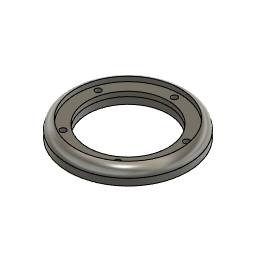
rear_speaker_adapter v3 (Autodesk Fusion 360 design; units mm, degrees)
Autodesk Fusion 360 part; units mm, degrees
note: some values were not read from the file. Chosen so that the rebuilt part matches the saved one: which face or edge a step refers to.
sketch "Sketch1" plane through (0, 0, 0) normal (0, 1, 0) x (1, 0, 0) in component "mounting ring"
  circle A0 centre (0, 0) radius 54
  circle A1 centre (0, 0) radius 36.5
  circle A2 centre (0, 0) radius 42
  circle A3 centre (0, 42) radius 2.625
  circle A4 centre (-39.9444, 12.9787) radius 2.625
  circle A5 centre (-24.687, -33.9787) radius 2.625
  circle A6 centre (24.687, -33.9787) radius 2.625
  circle A7 centre (39.9444, 12.9787) radius 2.625
  circle A8 centre (0, 0) radius 47.1
  line L0 (0, 0) -> (24.687, -33.9787)
  line L1 (0, 0) -> (-11.7659, -40.3183)
  line L2 (21.4542, -29.5291) -> (19.9517, -36.9585)
  line L3 (-10.2251, -35.0385) -> (-7.0236, -41.4086)
  dimension "d1" = 108
  dimension "d2" = 73
  dimension "d3" = 84
  dimension "d4" = 5.25
  dimension "d6" = 360
  dimension "d7" = 94.2
  dimension "d23" = 37
  constraint coincident A0.centre A1.centre
  constraint concentric A0 A1
  constraint coincident A2 A3.centre
  constraint concentric A1 A8
  constraint coincident A6.centre L0.end
  constraint coincident A2 L1.end
  constraint coincident A1 L2.start
  constraint coincident L0 L2.start
  constraint coincident A2 L2.end
  constraint coincident A1 L3.start
  constraint coincident L1 L3.start
  constraint coincident A2 L3.end
  measures "d1" diameter of A0
  measures "d2" diameter of A1
  measures "d3" diameter of A2
  measures "d4" diameter of A3
  measures "d7" diameter of A8
  measures "d23" distance of A6.centre L1.end
extrude "Extrude3" add sketch "Sketch1" along normal blind 8.5 contours A0 makes body 1 in component "mounting ring"
extrude "Extrude4" add sketch "Sketch1" along normal blind 4.25 contours A1 A2 A3 A4 A5 A6 A7 L0 L1 | A2 L1 L3 | A1 A2 L2 L3 | A2 A6 L0 L2 | A8 bodies 1 in component "mounting ring"
fillet "Fillet3" radius 8.68 1 edges at (-54, 8.5, 0) on bodies 1 in component "mounting ring"
extrude "Extrude5" add sketch "Sketch1" against normal blind 6 separate body contours A0 | A1 A2 A3 A4 A5 A6 A7 L0 L1 | A2 L1 L3 | A1 A2 L2 L3 | A2 A6 L0 L2 | A8 makes body 2 in component "mounting ring"
extrude "Extrude6" cut sketch "Sketch1" against normal up to surface (6 mm away) contours A1 A2 L2 L3 bodies 2 in component "mounting ring"
fillet "Fillet4" radius 15 2 edges at (21.4542, -3, 29.5291) (-10.2251, -3, 35.0385) on bodies 2 in component "mounting ring"
fillet "Fillet5" radius 5 2 edges at (19.9517, -3, 36.9585) (-7.0236, -3, 41.4086) on bodies 2 in component "mounting ring"
component "mounting ring" placed x (1, 0, 0) y (0, 1, 0) z (0, 0, 1) at (0, 0, 0)
named bodies: "Top", "Bottom"
